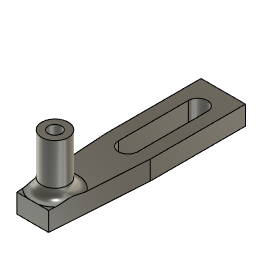
shaft_sa4_servo v2 (Autodesk Fusion 360 design; units mm, degrees)
Autodesk Fusion 360 part; units mm, degrees
note: some values were not read from the file. Set by a fixed rule: which sketch regions a step uses.
sketch "Sketch1" plane through (0, 0, 0) normal (0, 0, 1) x (1, 0, 0)
  line L0 (-10, 25) -> (-3, 25)
  line L1 (-3, 25) -> (-3, -5)
  line L2 (-3, -5) -> (-10, -5)
  line L3 (-10, -5) -> (-10, 25)
  line L4 (-10, -5) -> (-3, 2)
  line L5 (-10, -5) -> (-0.1005, -5) construction
  line L6 (-3, -5) -> (-10, 2)
  circle A0 centre (-6.5, -1.5) radius 2
  line L7 (-10, -5) -> (-9, -5)
  line L8 (-9, -5) -> (-10, 10)
  line L9 (-3, -5) -> (-4, -5)
  line L10 (-4, -5) -> (-3, 10)
  line L11 (-10, 25) -> (-3, 18)
  line L12 (-10, 25) -> (-0.1005, 25) construction
  line L13 (-3, 25) -> (-10, 18)
  line L14 (-6.5, 25) -> (-6.5, 22)
  line L15 (-6.5, 22) -> (-6.5, 9)
  line L16 (-5, 21) -> (-8, 21)
  line L17 (-8, 21) -> (-8, 10)
  line L18 (-8, 10) -> (-5, 10)
  line L19 (-5, 10) -> (-5, 21)
  line L20 (-5, 21) -> (-8, 10) construction
  line L21 (-8, 21) -> (-5, 10) construction
  circle A1 centre (-6.5, 10) radius 1.5
  circle A2 centre (-6.5, 21) radius 1.5
  point P0 (-6.5, 15.5)
  dimension "d1" = 7
  dimension "d2" = 30
  dimension "d3" = 45
  dimension "d4" = 4
  dimension "d5" = 45
  dimension "d6" = 3
  dimension "d7" = 13
  dimension "d8" = 3
  dimension "d9" = 11
  dimension "d10" = 3
  dimension "d11" = 3
  constraint horizontal L0
  constraint vertical L1
  constraint horizontal L2
  constraint vertical L3
  constraint horizontal L5
  constraint coincident L1 L4.end
  constraint coincident L3 L6.end
  constraint perpendicular L4 L6
  constraint midpoint L4 A0.centre
  constraint coincident L2 L7.end
  constraint midpoint L3 L8.end
  constraint coincident L2 L9.end
  constraint midpoint L1 L10.end
  constraint horizontal L12
  constraint coincident L1 L11.end
  constraint coincident L3 L13.end
  constraint perpendicular L11 L13
  constraint midpoint L0 L14.start
  constraint perpendicular L12 L14
  constraint parallel L3 L15
  constraint horizontal L16
  constraint perpendicular L16 L17
  constraint parallel L16 L18
  constraint parallel L17 L19
  constraint coincident L20 P0
  constraint coincident L21 P0
  constraint midpoint L15 P0
  constraint midpoint L18 A1.centre
  constraint midpoint L16 A2.centre
  measures "d1" distance of L0.start L0.end
  measures "d2" distance of L0.start L2.end
  measures "d3" angle of L4 L5
  measures "d4" diameter of A0
  measures "d5" angle of L11 L12
  measures "d6" distance of L14.start L14.end
  measures "d7" distance of L14.end L15.end
  measures "d8" distance of L17.end L18.end
  measures "d9" distance of L16.end L17.end
  measures "d10" diameter of A1
  measures "d11" diameter of A2
extrude "Extrude1" add sketch "Sketch1" along normal blind 2 contours L3 L11 L13 L17 A2 | L0 L11 L14 A2 | L0 L13 L14 A2 | L1 L3 L4 L6 A0 L8 L10 L11 L13 L17 L19 A1 | L1 L11 L13 L19 A2 | L4 L6 A0 L8 | L2 L4 L6 A0 L8 L10 | L4 L6 A0 L10
extrude "Extrude2" add sketch "Sketch1" along normal blind 10 contours L4 L6 A0 | L4 L6 A0 | L4 L6 A0 | L4 L6 A0
sketch "Sketch2" plane through (0, 0, 10) normal (0, 0, 1) x (-1, 0, 0)
  circle A0 centre (6.5, 1.5) radius 2
  circle A1 centre (6.5, 1.5) radius 1.05
  dimension "d16" = 2.1
  constraint concentric A0 A1
  measures "d16" diameter of A1
extrude "Extrude3" cut sketch "Sketch2" against normal blind 13 contours A1
move_face "OffsetFaces1" offset 0.1 1 faces at (-4.5025, -1.4003, 4.6667)
fillet "Fillet1" radius 1.5 1 edges at (-8.4579, -0.7406, 2)
extrude "Extrude4" add 1 faces at (-6.5374, 24.1653, 0) along direction (0, 0, -1) blind 1
